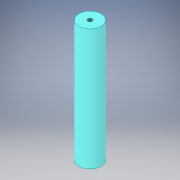
# Autodesk Inventor part: feet type 1 part 2
Saved by Autodesk Inventor 2018 (Build 220112000, 112)
## iProperties
Created: 2018-10-16
Part Number: feet type 1 part 2
Material: Fiber Glass
Document SubType Name: Modeling
Designer: freyja
Density: 1 g/cm^3
Appearance: Generic
Author: freyja
Autodesk Inventor part; units mm, degrees
ref_plane "YZ Plane" through (0, 0, 0) normal (1, 0, 0) x (0, 1, 0)
ref_plane "XZ Plane" through (0, 0, 0) normal (0, 1, 0) x (-1, 0, 0)
ref_plane "XY Plane" through (0, 0, 0) normal (0, 0, 1) x (1, 0, 0)
sketch "Sketch1" plane through (0, 0, 0) normal (0, 1, 0) x (-1, 0, 0)
  circle A0 centre (0, 0) radius 12.7
  dimension "d0" = 25.4
  constraints: 1 centre point, 1 coincident
  measures "d0" diameter of A0
extrude "Extrusion1" add sketch "Sketch1" along normal blind 139.1666
sketch "Sketch3" plane through (0, 139.1666, 0) normal (0, 1, 0) x (1, 0, 0)
  circle A0 centre (0, 0) radius 6.35
  dimension "d11" = 12.7
  constraints: 1 centre point, 1 coincident
  measures "d11" diameter of A0
sketch "Sketch2" plane through (0, 0, 0) normal (0, -1, 0) x (1, 0, 0)
  circle A0 centre (0, 0) radius 3.175
  dimension "d3" = 6.35
  constraints: 1 centre point, 1 coincident
  measures "d3" diameter of A0
hole "Hole1" at (0, 0, 0) direction (0, 1, 0) diameter 4.9784 depth 19.05 tip angle 118 thread size "1/4-20 UNC" class "2B" standard "ANSI Unified Screw Threads"
hole "Hole2" at (0, 139.1666, 0) direction (0, -1, 0) diameter 4.9784 depth 19.05 tip angle 118 thread size "1/4-20 UNC" class "2B" standard "ANSI Unified Screw Threads"
body "Solid1"
